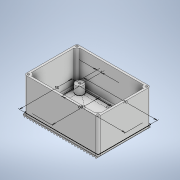
# Autodesk Inventor part: Enclosure
Saved by Autodesk Inventor 2020.2 (Build 242310000, 310)
## iProperties
Created: 2020-09-23
Part Number: Enclosure
Material: Generic
Document SubType Name: Modeling
Designer: johnf
Density: 1 g/cm^3
Appearance: Default
Author: johnf
Autodesk Inventor part; units mm, degrees
ref_plane "YZ Plane" through (0, 0, 0) normal (1, 0, 0) x (0, 1, 0)
ref_plane "XZ Plane" through (0, 0, 0) normal (0, 1, 0) x (-1, 0, 0)
ref_plane "XY Plane" through (0, 0, 0) normal (0, 0, 1) x (1, 0, 0)
sketch "Sketch1" plane through (0, 0, 0) normal (0, 1, 0) x (-1, 0, 0)
  line L0 (25, 17.5) -> (-25, 17.5) construction
  line L1 (-25, 17.5) -> (-25, -17.5) construction
  line L2 (-25, -17.5) -> (25, -17.5) construction
  line L3 (25, -17.5) -> (25, 17.5) construction
  line L4 (25, -17.5) -> (-25, 17.5) construction
  circle A0 centre (25, 17.5) radius 1
  circle A1 centre (25, -17.5) radius 1
  circle A2 centre (-25, 17.5) radius 1
  circle A3 centre (-25, -17.5) radius 1
  circle A4 centre (25, 17.5) radius 3.75
  circle A5 centre (25, -17.5) radius 3.75
  circle A6 centre (-25, -17.5) radius 3.75
  circle A7 centre (-25, 17.5) radius 3.75
  point P0 (0, 0)
  point P1 (0, 0)
  dimension "d0" = 35
  dimension "d1" = 50
  dimension "d2" = 2
  dimension "d3" = 7.5
  constraints: 10 end point, 9 coincident, 8 centre point, 6 equal radius, 2 parallel, 1 horizontal, 1 midpoint, 1 perpendicular
  measures "d0" distance of L2.end L0.start
  measures "d1" distance of L1.end L2.end
  measures "d2" diameter of A0
  measures "d3" diameter of A4
extrude "Extrusion1" add sketch "Sketch1" along normal blind 7.5
sketch "Sketch2" plane through (0, 0, 0) normal (0, 1, 0) x (-1, 0, 0)
  line L0 (35, -25) -> (-35, -25)
  line L1 (-35, -25) -> (-35, 25)
  line L2 (-35, 25) -> (35, 25)
  line L3 (35, 25) -> (35, -25)
  line L4 (35, 25) -> (-35, -25) construction
  line L5 (30, -22.5) -> (-30, -22.5) construction
  line L6 (-30, -22.5) -> (-30, 22.5) construction
  line L7 (-30, 22.5) -> (30, 22.5) construction
  line L8 (30, 22.5) -> (30, -22.5) construction
  line L9 (-25, -17.5) -> (25, -17.5) construction
  line L10 (25, -17.5) -> (25, 17.5) construction
  line L11 (25, 17.5) -> (-25, 17.5) construction
  line L12 (-25, 17.5) -> (-25, -17.5) construction
  line L13 (30, -22.5) -> (-30, 22.5) construction
  line L14 (-31, -21) -> (31, -21)
  line L15 (31, -21) -> (31, 21)
  line L16 (31, 21) -> (-31, 21)
  line L17 (-31, 21) -> (-31, -21)
  circle A0 centre (25, -17.5) radius 3.75
  circle A1 centre (-25, -17.5) radius 1 projected
  circle A2 centre (-25, -17.5) radius 3.75
  circle A3 centre (-25, 17.5) radius 3.75
  circle A4 centre (25, 17.5) radius 3.75
  circle A5 centre (25, -17.5) radius 3.75 projected
  circle A6 centre (25, 17.5) radius 3.75 projected
  circle A7 centre (-25, 17.5) radius 3.75 projected
  point P0 (0, 0)
  point P1 (0, 0)
  dimension "d6" = 70
  dimension "d7" = 60
  dimension "d8" = 45
  dimension "d9" = 5
  dimension "d10" = 50
  dimension "d11" = 4
  constraints: 36 end point, 8 parallel, 5 coincident, 4 centre point, 4 equal radius, 4 perpendicular, 2 horizontal, 2 midpoint, 6 other
  measures "d6" distance of L0.start L0.end
  measures "d7" distance of L5.start L5.end
  measures "d8" distance of L7.end L5.start
  measures "d9" distance between parallel lines of L5 L9
  measures "d10" distance of L2.end L0.start
  measures "d11" distance between parallel lines of L3 L15
extrude "Extrusion2" add sketch "Sketch2" against normal blind 2 contours L0 L1 L2 L3 | L17 L16 A3 A4 L15 L14 A0 A2 | A2 L14 | L14 A2 | A3 L16 | L16 A3 | A0 L14 | L14 A0 | A4 L16 | L16 A4 | A1
extrude "Extrusion3" add sketch "Sketch2" along normal blind 1 contours L0 L1 L2 L3 | L14 A2 | A3 L16 | L14 A0 | A4 L16 picked at (-24.8474, -21.074) picked at (-24.8474, 21.074) picked at (25.1526, -21.074) picked at (24.8474, 21.074)
sketch "Sketch5" plane through (0, 1, 0) normal (0, 1, 0) x (1, 0, 0)
  line L0 (-35, -25) -> (-35, 25) projected
  line L1 (35, 25) -> (35, -25) projected
  line L2 (-35, 25) -> (35, 25)
  line L3 (35, 25) -> (35, -25)
  line L4 (35, -25) -> (-35, -25)
  line L5 (-35, -25) -> (-35, 25)
  line L6 (30.1716, 23) -> (-30.1716, 23)
  line L7 (-33, 20.1716) -> (-33, -20.1716)
  line L8 (-30.1716, -23) -> (30.1716, -23)
  line L9 (33, -20.1716) -> (33, 20.1716)
  line L10 (-31, 21) -> (-31, -21) projected
  arc A0 (-30.1716, -23) -> (-33, -20.1716) centre (-33, -23) ccw
  line L11 (31, 21) -> (31, -21) projected
  arc A1 (-33, 20.1716) -> (-30.1716, 23) centre (-33, 23) ccw
  arc A2 (33, -20.1716) -> (30.1716, -23) centre (33, -23) ccw
  arc A3 (30.1716, 23) -> (33, 20.1716) centre (33, 23) ccw
  point P0 (0, 0)
  point P1 (-35, -25)
  dimension "d17" = 2
  dimension "d20" = 2
  dimension "d21" = 2
  dimension "d22" = 2.8284
  dimension "d23" = 2
  constraints: 16 end point, 12 point on circle, 7 point on line, 4 centre point, 4 parallel, 2 perpendicular, 1 horizontal
  measures "d17" distance between parallel lines of L2 L6
  measures "d20" distance between parallel lines of L0 L7
  measures "d21" distance between parallel lines of L3 L9
  measures "d22" radius of A3
  measures "d23" distance between parallel lines of L4 L8
extrude "Extrusion4" add sketch "Sketch5" along normal blind 30
sketch "Sketch6" plane through (0, 31, 0) normal (0, 1, 0) x (1, 0, 0)
  circle A0 centre (-33, 23) radius 1
  line L0 (-30.1716, 23) -> (30.1716, 23) projected
  line L1 (-33, -20.1716) -> (-33, 20.1716) projected
  circle A1 centre (33, 23) radius 1
  circle A2 centre (33, -23) radius 1
  circle A3 centre (-33, -23) radius 1
  line L2 (33, 20.1716) -> (33, -20.1716) projected
  line L3 (30.1716, -23) -> (-30.1716, -23) projected
  point P0 (0, 0)
  dimension "d24" = 2
  constraints: 8 point on line, 4 centre point, 3 equal radius
  measures "d24" diameter of A0
extrude "Extrusion5" cut sketch "Sketch6" against normal blind 10
fillet "Fillet1" radius 2 4 edges at (-35, 14.5, -25) (35, 14.5, -25) (35, 14.5, 25) (-35, 14.5, 25)
sketch "Sketch7" plane through (33, -2, -25) normal (0, 0, -1) x (-1, 0, 0)
  line L0 (-2, -0.25) -> (0, -2.25)
  line L1 (0, -2.25) -> (1.4142, -0.8358)
  line L2 (-2, -0.25) -> (68, -0.25)
  line L3 (66, 0) -> (0, 0) projected
  line L4 (-2, 33) -> (-2, 0) projected
  line L5 (0, 0) -> (-2, 0) projected
  line L6 (1.4142, -0.8358) -> (2.8284, -2.25)
  line L7 (2.8284, -2.25) -> (4.2426, -0.8358)
  line L8 (4.2426, -0.8358) -> (5.6569, -2.25)
  line L9 (5.6569, -2.25) -> (7.0711, -0.8358)
  line L10 (7.0711, -0.8358) -> (8.4853, -2.25)
  line L11 (8.4853, -2.25) -> (9.8995, -0.8358)
  line L12 (9.8995, -0.8358) -> (11.3137, -2.25)
  line L13 (11.3137, -2.25) -> (12.7279, -0.8358)
  line L14 (12.7279, -0.8358) -> (14.1421, -2.25)
  line L15 (14.1421, -2.25) -> (15.5563, -0.8358)
  line L16 (15.5563, -0.8358) -> (16.9706, -2.25)
  line L17 (16.9706, -2.25) -> (18.3848, -0.8358)
  line L18 (18.3848, -0.8358) -> (19.799, -2.25)
  line L19 (19.799, -2.25) -> (21.2132, -0.8358)
  line L20 (21.2132, -0.8358) -> (22.6274, -2.25)
  line L21 (22.6274, -2.25) -> (24.0416, -0.8358)
  line L22 (24.0416, -0.8358) -> (25.4558, -2.25)
  line L23 (25.4558, -2.25) -> (26.8701, -0.8358)
  line L24 (26.8701, -0.8358) -> (28.2843, -2.25)
  line L25 (28.2843, -2.25) -> (29.6985, -0.8358)
  line L26 (29.6985, -0.8358) -> (31.1127, -2.25)
  line L27 (31.1127, -2.25) -> (32.5269, -0.8358)
  line L28 (32.5269, -0.8358) -> (33.9411, -2.25)
  line L29 (33.9411, -2.25) -> (35.3553, -0.8358)
  line L30 (36.7696, -2.25) -> (38.1838, -0.8358)
  line L31 (38.1838, -0.8358) -> (39.598, -2.25)
  line L32 (39.598, -2.25) -> (41.0122, -0.8358)
  line L33 (41.0122, -0.8358) -> (42.4264, -2.25)
  line L34 (42.4264, -2.25) -> (43.8406, -0.8358)
  line L35 (43.8406, -0.8358) -> (45.2548, -2.25)
  line L36 (35.3553, -0.8358) -> (36.7696, -2.25)
  line L37 (45.2548, -2.25) -> (46.669, -0.8358)
  line L38 (46.669, -0.8358) -> (48.0833, -2.25)
  line L39 (48.0833, -2.25) -> (49.4975, -0.8358)
  line L40 (49.4975, -0.8358) -> (50.9117, -2.25)
  line L41 (50.9117, -2.25) -> (52.3259, -0.8358)
  line L42 (52.3259, -0.8358) -> (53.7401, -2.25)
  line L43 (53.7401, -2.25) -> (55.1543, -0.8358)
  line L44 (56.5685, -2.25) -> (57.9828, -0.8358)
  line L45 (57.9828, -0.8358) -> (59.397, -2.25)
  line L46 (59.397, -2.25) -> (60.8112, -0.8358)
  line L47 (60.8112, -0.8358) -> (62.2254, -2.25)
  line L48 (62.2254, -2.25) -> (63.6396, -0.8358)
  line L49 (63.6396, -0.8358) -> (65.0538, -2.25)
  line L50 (55.1543, -0.8358) -> (56.5685, -2.25)
  line L51 (65.0538, -2.25) -> (66.468, -0.8358)
  line L52 (66.468, -0.8358) -> (67.8823, -2.25)
  line L53 (68, -0.25) -> (69.1812, -0.25)
  line L54 (69.1812, -0.25) -> (67.8823, -2.25)
  point P0 (33, 2)
  dimension "d29" = 2
  dimension "d30" = 70
  dimension "d31" = 0.25
  dimension "d32" = 90
  dimension "d33" = 45
  dimension "d34" = 90
  dimension "d35" = 2
  dimension "d36" = 90
  dimension "d37" = 2
  dimension "d38" = 90
  dimension "d39" = 90
  dimension "d40" = 2
  dimension "d41" = 90
  dimension "d42" = 2
  dimension "d43" = 90
  dimension "d44" = 90
  dimension "d45" = 90
  dimension "d46" = 2
  dimension "d47" = 90
  dimension "d48" = 2
  dimension "d49" = 90
  dimension "d50" = 90
  dimension "d51" = 2
  dimension "d52" = 90
  dimension "d53" = 2
  dimension "d54" = 90
  dimension "d55" = 90
  dimension "d56" = 90
  dimension "d57" = 90
  dimension "d58" = 2
  dimension "d59" = 90
  dimension "d60" = 2
  dimension "d61" = 90
  dimension "d62" = 90
  dimension "d63" = 2
  dimension "d64" = 90
  dimension "d65" = 2
  dimension "d66" = 90
  dimension "d67" = 90
  dimension "d68" = 90
  dimension "d69" = 2
  dimension "d70" = 90
  dimension "d71" = 2
  dimension "d72" = 90
  dimension "d73" = 90
  dimension "d74" = 2
  dimension "d75" = 90
  dimension "d76" = 2
  dimension "d77" = 90
  dimension "d78" = 90
  dimension "d79" = 90
  dimension "d81" = 90
  dimension "d82" = 90
  dimension "d83" = 2
  dimension "d84" = 90
  dimension "d85" = 2
  dimension "d86" = 90
  dimension "d87" = 2
  dimension "d88" = 90
  dimension "d89" = 90
  dimension "d90" = 90
  dimension "d91" = 2
  dimension "d92" = 90
  dimension "d93" = 2
  constraints: 104 end point, 24 perpendicular, 1 horizontal, 1 parallel, 1 point on line
  measures "d29" horizontal distance of L0.start L0.end
  measures "d30" distance of L0.start L2.end
  measures "d31" distance between parallel lines of L5 L2
  measures "d32" angle of L1 L6
  measures "d33" angle of L2 L0
  measures "d34" angle of L0 L1
  measures "d35" distance of L0.end L1.end
  measures "d36" angle of L7 L8
  measures "d37" distance of L6.end L7.end
  measures "d38" angle of L6 L7
  measures "d39" angle of L9 L10
  measures "d40" distance of L8.end L9.end
  measures "d41" angle of L11 L12
  measures "d42" distance of L10.end L11.end
  measures "d43" angle of L10 L11
  measures "d44" angle of L8 L9
  measures "d45" angle of L13 L14
  measures "d46" distance of L12.end L13.end
  measures "d47" angle of L15 L16
  measures "d48" distance of L15.start L15.end
  measures "d49" angle of L14 L15
  measures "d50" angle of L17 L18
  measures "d51" distance of L16.end L17.end
  measures "d52" angle of L19 L20
  measures "d53" distance of L18.end L19.end
  measures "d54" angle of L18 L19
  measures "d55" angle of L16 L17
  measures "d56" angle of L12 L13
  measures "d57" angle of L21 L22
  measures "d58" distance of L20.end L21.end
  measures "d59" angle of L23 L24
  measures "d60" distance of L23.start L24.start
  measures "d61" angle of L22 L23
  measures "d62" angle of L25 L26
  measures "d63" distance of L25.start L26.start
  measures "d64" angle of L27 L28
  measures "d65" distance of L27.start L28.start
  measures "d66" angle of L26 L27
  measures "d67" angle of L24 L25
  measures "d68" angle of L29 L36
  measures "d69" distance of L29.start L36.start
  measures "d70" angle of L30 L31
  measures "d71" distance of L30.start L31.start
  measures "d72" angle of L36 L30
  measures "d73" angle of L32 L33
  measures "d74" distance of L32.start L33.start
  measures "d75" angle of L34 L35
  measures "d76" distance of L34.start L34.end
  measures "d77" angle of L33 L34
  measures "d78" angle of L31 L32
  measures "d79" angle of L28 L29
  measures "d81" angle of L20 L21
  measures "d82" angle of L37 L38
  measures "d83" distance of L35.end L38.start
  measures "d84" angle of L39 L40
  measures "d85" distance of L39.start L39.end
  measures "d86" angle of L41 L42
  measures "d87" distance of L40.end L41.end
  measures "d88" angle of L40 L41
  measures "d89" angle of L38 L39
  measures "d90" angle of L43 L50
  measures "d91" distance of L42.end L43.end
  measures "d92" angle of L44 L45
  measures "d93" distance of L50.end L44.end
extrude "Extrusion6" add sketch "Sketch7" against normal up to surface (50 mm away)
body "Solid1"
